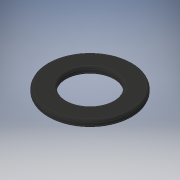
# Autodesk Inventor part: ruela m6 borracha
Saved by Autodesk Inventor 2019.4 (Build 234330000, 330)
## iProperties
Created: 2021-02-09
Part Number: ruela m6 borracha
Material: Borracha
Document SubType Name: Modeling
Designer: Lattes
Density: 0.93 g/cm^3
Appearance: Borracha - Preta
Author: Lattes
Autodesk Inventor part; units mm, degrees
ref_plane "YZ Plane" through (0, 0, 0) normal (1, 0, 0) x (0, 1, 0)
ref_plane "XZ Plane" through (0, 0, 0) normal (0, 1, 0) x (-1, 0, 0)
ref_plane "XY Plane" through (0, 0, 0) normal (0, 0, 1) x (1, 0, 0)
sketch "Esboço1" plane through (0, 0, 0) normal (0, 1, 0) x (-1, 0, 0)
  circle A0 centre (0, 0) radius 3.5
  circle A1 centre (0, 0) radius 6.25
  dimension "d0" = 7
  dimension "d1" = 12.5
  constraints: 2 centre point, 2 coincident
  measures "d0" diameter of A0
  measures "d1" diameter of A1
extrude "Extrusão1" add sketch "Esboço1" along normal blind 1
fillet "Arredondamento1" radius 0.3 4 edges at (3.5, 1, 0) (6.25, 1, 0) (3.5, 0, 0) (6.25, 0, 0)
